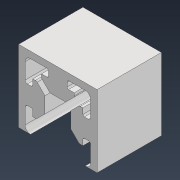
# Autodesk Inventor part: Part6
Saved by Autodesk Inventor 2022 (Build 260153000, 153)
## iProperties
Created: 2022-06-24
Part Number: Part6
Material: Generic
Document SubType Name: Modeling
Designer: tecware
Density: 1 g/cm^3
Appearance: Default
Author: tecware
Autodesk Inventor part; units mm, degrees
ref_plane "YZ Plane" through (0, 0, 0) normal (1, 0, 0) x (0, 1, 0)
ref_plane "XZ Plane" through (0, 0, 0) normal (0, 1, 0) x (-1, 0, 0)
ref_plane "XY Plane" through (0, 0, 0) normal (0, 0, 1) x (1, 0, 0)
sketch "Sketch1" plane through (0, 0, 0) normal (0, 0, 1) x (1, 0, 0)
  arc A0 (-1.0546, 0.6324) -> (-0.3475, 0.9253) centre (-1.0546, 1.6324) ccw projected
  line L0 (-1.0546, 0.6324) -> (-1.8676, 0.6324) projected
  arc A1 (-2.0676, 0.8324) -> (-1.8676, 0.6324) centre (-1.8676, 0.8324) ccw projected
  line L1 (-2.0676, 0.8324) -> (-2.0676, 2.6024) projected
  arc A2 (-2.0676, 2.6024) -> (-2.3176, 2.8524) centre (-2.3176, 2.6024) ccw projected
  line L2 (-2.3176, 2.8524) -> (-3.5676, 2.8524) projected
  arc A3 (-3.5676, 2.8524) -> (-4.0676, 2.3524) centre (-3.5676, 2.3524) ccw projected
  line L3 (-4.0676, 2.3524) -> (-4.0676, -2.5676) projected
  arc A4 (-4.0676, -2.5676) -> (-2.5676, -4.0676) centre (-2.5676, -2.5676) ccw projected
  line L4 (-2.5676, -4.0676) -> (2.3524, -4.0676) projected
  arc A5 (2.3524, -4.0676) -> (2.8524, -3.5676) centre (2.3524, -3.5676) ccw projected
  line L5 (2.8524, -3.5676) -> (2.8524, -2.3176) projected
  arc A6 (2.8524, -2.3176) -> (2.6024, -2.0676) centre (2.6024, -2.3176) ccw projected
  line L6 (2.6024, -2.0676) -> (0.8324, -2.0676) projected
  arc A7 (0.6324, -1.8676) -> (0.8324, -2.0676) centre (0.8324, -1.8676) ccw projected
  line L7 (0.6324, -1.8676) -> (0.6324, -1.0546) projected
  arc A8 (0.9253, -0.3475) -> (0.6324, -1.0546) centre (1.6324, -1.0546) ccw projected
  line L8 (0.9253, -0.3475) -> (4.0676, 2.7948) projected
  arc A9 (4.0676, 2.7948) -> (5.6798, 2.2912) centre (5.9324, 5.9324) ccw projected
  line L9 (5.6798, 2.2912) -> (5.9324, 2.491) projected
  line L10 (5.9324, 2.491) -> (6.1851, 2.2912) projected
  arc A10 (6.1851, 2.2912) -> (7.7973, 2.7948) centre (5.9324, 5.9324) ccw projected
  line L11 (7.7973, 2.7948) -> (10.9395, -0.3475) projected
  arc A11 (11.2324, -1.0546) -> (10.9395, -0.3475) centre (10.2324, -1.0546) ccw projected
  line L12 (11.2324, -1.0546) -> (11.2324, -1.8676) projected
  arc A12 (11.0324, -2.0676) -> (11.2324, -1.8676) centre (11.0324, -1.8676) ccw projected
  line L13 (11.0324, -2.0676) -> (9.2624, -2.0676) projected
  arc A13 (9.2624, -2.0676) -> (9.0124, -2.3176) centre (9.2624, -2.3176) ccw projected
  line L14 (9.0124, -2.3176) -> (9.0124, -3.5676) projected
  arc A14 (9.0124, -3.5676) -> (9.5124, -4.0676) centre (9.5124, -3.5676) ccw projected
  line L15 (9.5124, -4.0676) -> (14.4324, -4.0676) projected
  arc A15 (14.4324, -4.0676) -> (15.9324, -2.5676) centre (14.4324, -2.5676) ccw projected
  line L16 (15.9324, -2.5676) -> (15.9324, 2.3524) projected
  arc A16 (15.9324, 2.3524) -> (15.4324, 2.8524) centre (15.4324, 2.3524) ccw projected
  line L17 (15.4324, 2.8524) -> (14.1824, 2.8524) projected
  arc A17 (14.1824, 2.8524) -> (13.9324, 2.6024) centre (14.1824, 2.6024) ccw projected
  line L18 (13.9324, 2.6024) -> (13.9324, 0.8324) projected
  arc A18 (13.7324, 0.6324) -> (13.9324, 0.8324) centre (13.7324, 0.8324) ccw projected
  line L19 (13.7324, 0.6324) -> (12.9194, 0.6324) projected
  arc A19 (12.2123, 0.9253) -> (12.9194, 0.6324) centre (12.9194, 1.6324) ccw projected
  line L20 (12.2123, 0.9253) -> (9.0701, 4.0676) projected
  arc A20 (9.0701, 4.0676) -> (9.5737, 5.6798) centre (5.9324, 5.9324) ccw projected
  line L21 (9.5737, 5.6798) -> (9.3739, 5.9324) projected
  line L22 (9.3739, 5.9324) -> (9.5739, 6.1824) projected
  arc A21 (9.5739, 6.1824) -> (9.0701, 7.7973) centre (5.9324, 5.9324) ccw projected
  line L23 (9.0701, 7.7973) -> (12.2123, 10.9395) projected
  arc A22 (12.9194, 11.2324) -> (12.2123, 10.9395) centre (12.9194, 10.2324) ccw projected
  line L24 (12.9194, 11.2324) -> (13.7324, 11.2324) projected
  arc A23 (13.9324, 11.0324) -> (13.7324, 11.2324) centre (13.7324, 11.0324) ccw projected
  line L25 (13.9324, 11.0324) -> (13.9324, 9.2624) projected
  arc A24 (13.9324, 9.2624) -> (14.1824, 9.0124) centre (14.1824, 9.2624) ccw projected
  line L26 (14.1824, 9.0124) -> (15.4324, 9.0124) projected
  arc A25 (15.4324, 9.0124) -> (15.9324, 9.5124) centre (15.4324, 9.5124) ccw projected
  line L27 (15.9324, 9.5124) -> (15.9324, 14.4324) projected
  arc A26 (15.9324, 14.4324) -> (14.4324, 15.9324) centre (14.4324, 14.4324) ccw projected
  line L28 (14.4324, 15.9324) -> (9.5124, 15.9324) projected
  arc A27 (9.5124, 15.9324) -> (9.0124, 15.4324) centre (9.5124, 15.4324) ccw projected
  line L29 (9.0124, 15.4324) -> (9.0124, 14.1824) projected
  arc A28 (9.0124, 14.1824) -> (9.2624, 13.9324) centre (9.2624, 14.1824) ccw projected
  line L30 (9.2624, 13.9324) -> (11.0324, 13.9324) projected
  arc A29 (11.2324, 13.7324) -> (11.0324, 13.9324) centre (11.0324, 13.7324) ccw projected
  line L31 (11.2324, 13.7324) -> (11.2324, 12.9194) projected
  arc A30 (10.9395, 12.2123) -> (11.2324, 12.9194) centre (10.2324, 12.9194) ccw projected
  line L32 (10.9395, 12.2123) -> (7.7973, 9.0701) projected
  arc A31 (7.7973, 9.0701) -> (6.1824, 9.5739) centre (5.9324, 5.9324) ccw projected
  line L33 (6.1824, 9.5739) -> (5.9324, 9.3739) projected
  line L34 (5.9324, 9.3739) -> (5.6824, 9.5739) projected
  arc A32 (5.6824, 9.5739) -> (4.0676, 9.0701) centre (5.9324, 5.9324) ccw projected
  line L35 (4.0676, 9.0701) -> (0.9253, 12.2123) projected
  arc A33 (0.6324, 12.9194) -> (0.9253, 12.2123) centre (1.6324, 12.9194) ccw projected
  line L36 (0.6324, 12.9194) -> (0.6324, 13.7324) projected
  arc A34 (0.8324, 13.9324) -> (0.6324, 13.7324) centre (0.8324, 13.7324) ccw projected
  line L37 (0.8324, 13.9324) -> (2.6024, 13.9324) projected
  arc A35 (2.6024, 13.9324) -> (2.8524, 14.1824) centre (2.6024, 14.1824) ccw projected
  line L38 (2.8524, 14.1824) -> (2.8524, 15.4324) projected
  arc A36 (2.8524, 15.4324) -> (2.3524, 15.9324) centre (2.3524, 15.4324) ccw projected
  line L39 (2.3524, 15.9324) -> (-2.5676, 15.9324) projected
  arc A37 (-2.5676, 15.9324) -> (-4.0676, 14.4324) centre (-2.5676, 14.4324) ccw projected
  line L40 (-4.0676, 14.4324) -> (-4.0676, 9.5124) projected
  arc A38 (-4.0676, 9.5124) -> (-3.5676, 9.0124) centre (-3.5676, 9.5124) ccw projected
  line L41 (-3.5676, 9.0124) -> (-2.3176, 9.0124) projected
  arc A39 (-2.3176, 9.0124) -> (-2.0676, 9.2624) centre (-2.3176, 9.2624) ccw projected
  line L42 (-2.0676, 9.2624) -> (-2.0676, 11.0324) projected
  arc A40 (-1.8676, 11.2324) -> (-2.0676, 11.0324) centre (-1.8676, 11.0324) ccw projected
  line L43 (-1.8676, 11.2324) -> (-1.0546, 11.2324) projected
  arc A41 (-0.3475, 10.9395) -> (-1.0546, 11.2324) centre (-1.0546, 10.2324) ccw projected
  line L44 (-0.3475, 10.9395) -> (2.7948, 7.7973) projected
  arc A42 (2.7948, 7.7973) -> (2.291, 6.1824) centre (5.9324, 5.9324) ccw projected
  line L45 (2.291, 6.1824) -> (2.491, 5.9324) projected
  line L46 (2.491, 5.9324) -> (2.2912, 5.6798) projected
  arc A43 (2.2912, 5.6798) -> (2.7948, 4.0676) centre (5.9324, 5.9324) ccw projected
  line L47 (2.7948, 4.0676) -> (-0.3475, 0.9253) projected
  circle A44 centre (5.9324, 5.9324) radius 2.5 projected
  line L48 (-1.0546, 11.0324) -> (-1.8676, 11.0324)
  line L49 (-1.8676, 11.0324) -> (-1.8676, 9.2624)
  arc A45 (-2.3176, 8.8124) -> (-1.8676, 9.2624) centre (-2.3176, 9.2624) ccw
  line L50 (-2.3176, 8.8124) -> (-3.5676, 8.8124)
  arc A46 (-4.2676, 9.5124) -> (-3.5676, 8.8124) centre (-3.5676, 9.5124) ccw
  line L51 (-4.2676, 9.5124) -> (-4.2676, 14.4324)
  arc A47 (-2.5676, 16.1324) -> (-4.2676, 14.4324) centre (-2.5676, 14.4324) ccw
  line L52 (-2.5676, 16.1324) -> (2.3524, 16.1324)
  arc A48 (3.0524, 15.4324) -> (2.3524, 16.1324) centre (2.3524, 15.4324) ccw
  line L53 (3.0524, 15.4324) -> (3.0524, 14.1824)
  arc A49 (2.6024, 13.7324) -> (3.0524, 14.1824) centre (2.6024, 14.1824) ccw
  line L54 (2.6024, 13.7324) -> (0.8324, 13.7324)
  line L55 (0.8324, 13.7324) -> (0.8324, 12.9194)
  arc A50 (0.8324, 12.9194) -> (1.0667, 12.3537) centre (1.6324, 12.9194) ccw
  line L56 (1.0667, 12.3537) -> (4.1014, 9.3191)
  arc A51 (5.7474, 9.778) -> (4.1014, 9.3191) centre (5.9324, 5.9324) ccw
  line L57 (5.7474, 9.778) -> (5.9324, 9.63)
  line L58 (5.9324, 9.63) -> (6.1174, 9.778)
  arc A52 (7.7635, 9.3191) -> (6.1174, 9.778) centre (5.9324, 5.9324) ccw
  line L59 (7.7635, 9.3191) -> (10.7981, 12.3537)
  arc A53 (10.7981, 12.3537) -> (11.0324, 12.9194) centre (10.2324, 12.9194) ccw
  line L60 (11.0324, 12.9194) -> (11.0324, 13.7324)
  line L61 (11.0324, 13.7324) -> (9.2624, 13.7324)
  arc A54 (8.8124, 14.1824) -> (9.2624, 13.7324) centre (9.2624, 14.1824) ccw
  line L62 (8.8124, 14.1824) -> (8.8124, 15.4324)
  arc A55 (9.5124, 16.1324) -> (8.8124, 15.4324) centre (9.5124, 15.4324) ccw
  line L63 (9.5124, 16.1324) -> (14.4324, 16.1324)
  arc A56 (16.1324, 14.4324) -> (14.4324, 16.1324) centre (14.4324, 14.4324) ccw
  line L64 (16.1324, 14.4324) -> (16.1324, 9.5124)
  arc A57 (15.4324, 8.8124) -> (16.1324, 9.5124) centre (15.4324, 9.5124) ccw
  line L65 (15.4324, 8.8124) -> (14.1824, 8.8124)
  arc A58 (13.7324, 9.2624) -> (14.1824, 8.8124) centre (14.1824, 9.2624) ccw
  line L66 (13.7324, 9.2624) -> (13.7324, 11.0324)
  line L67 (13.7324, 11.0324) -> (12.9194, 11.0324)
  arc A59 (12.9194, 11.0324) -> (12.3537, 10.7981) centre (12.9194, 10.2324) ccw
  line L68 (12.3537, 10.7981) -> (9.3191, 7.7635)
  arc A60 (9.778, 6.1174) -> (9.3191, 7.7635) centre (5.9324, 5.9324) ccw
  line L69 (9.778, 6.1174) -> (9.6294, 5.9317)
  line L70 (9.6294, 5.9317) -> (9.7778, 5.7441)
  arc A61 (9.3191, 4.1014) -> (9.7778, 5.7441) centre (5.9324, 5.9324) ccw
  line L71 (9.3191, 4.1014) -> (12.3537, 1.0667)
  arc A62 (12.3537, 1.0667) -> (12.9194, 0.8324) centre (12.9194, 1.6324) ccw
  line L72 (12.9194, 0.8324) -> (13.7324, 0.8324)
  line L73 (13.7324, 0.8324) -> (13.7324, 2.6024)
  arc A63 (14.1824, 3.0524) -> (13.7324, 2.6024) centre (14.1824, 2.6024) ccw
  line L74 (14.1824, 3.0524) -> (15.4324, 3.0524)
  arc A64 (16.1324, 2.3524) -> (15.4324, 3.0524) centre (15.4324, 2.3524) ccw
  line L75 (16.1324, 2.3524) -> (16.1324, -2.5676)
  arc A65 (14.4324, -4.2676) -> (16.1324, -2.5676) centre (14.4324, -2.5676) ccw
  line L76 (14.4324, -4.2676) -> (9.5124, -4.2676)
  arc A66 (8.8124, -3.5676) -> (9.5124, -4.2676) centre (9.5124, -3.5676) ccw
  line L77 (8.8124, -3.5676) -> (8.8124, -2.3176)
  arc A67 (9.2624, -1.8676) -> (8.8124, -2.3176) centre (9.2624, -2.3176) ccw
  line L78 (9.2624, -1.8676) -> (11.0324, -1.8676)
  line L79 (11.0324, -1.8676) -> (11.0324, -1.0546)
  arc A68 (11.0324, -1.0546) -> (10.7981, -0.4889) centre (10.2324, -1.0546) ccw
  line L80 (10.7981, -0.4889) -> (7.7635, 2.5457)
  arc A69 (6.1208, 2.087) -> (7.7635, 2.5457) centre (5.9324, 5.9324) ccw
  line L81 (6.1208, 2.087) -> (5.9324, 2.236)
  line L82 (5.9324, 2.236) -> (5.7441, 2.087)
  arc A70 (4.1014, 2.5457) -> (5.7441, 2.087) centre (5.9324, 5.9324) ccw
  line L83 (4.1014, 2.5457) -> (1.0667, -0.4889)
  arc A71 (1.0667, -0.4889) -> (0.8324, -1.0546) centre (1.6324, -1.0546) ccw
  line L84 (0.8324, -1.0546) -> (0.8324, -1.8676)
  line L85 (0.8324, -1.8676) -> (2.6024, -1.8676)
  arc A72 (3.0524, -2.3176) -> (2.6024, -1.8676) centre (2.6024, -2.3176) ccw
  line L86 (3.0524, -2.3176) -> (3.0524, -3.5676)
  arc A73 (2.3524, -4.2676) -> (3.0524, -3.5676) centre (2.3524, -3.5676) ccw
  line L87 (2.3524, -4.2676) -> (-2.5676, -4.2676)
  arc A74 (-4.2676, -2.5676) -> (-2.5676, -4.2676) centre (-2.5676, -2.5676) ccw
  line L88 (-4.2676, -2.5676) -> (-4.2676, 2.3524)
  arc A75 (-3.5676, 3.0524) -> (-4.2676, 2.3524) centre (-3.5676, 2.3524) ccw
  line L89 (-3.5676, 3.0524) -> (-2.3176, 3.0524)
  arc A76 (-1.8676, 2.6024) -> (-2.3176, 3.0524) centre (-2.3176, 2.6024) ccw
  line L90 (-1.8676, 2.6024) -> (-1.8676, 0.8324)
  line L91 (-1.8676, 0.8324) -> (-1.0546, 0.8324)
  arc A77 (-1.0546, 0.8324) -> (-0.4889, 1.0667) centre (-1.0546, 1.6324) ccw
  line L92 (-0.4889, 1.0667) -> (2.5457, 4.1014)
  arc A78 (2.087, 5.7441) -> (2.5457, 4.1014) centre (5.9324, 5.9324) ccw
  line L93 (2.087, 5.7441) -> (2.2354, 5.9317)
  line L94 (2.2354, 5.9317) -> (2.0869, 6.1174)
  arc A79 (2.5457, 7.7635) -> (2.0869, 6.1174) centre (5.9324, 5.9324) ccw
  line L95 (2.5457, 7.7635) -> (-0.4889, 10.7981)
  arc A80 (-0.4889, 10.7981) -> (-1.0546, 11.0324) centre (-1.0546, 10.2324) ccw
  line L96 (-4.2676, -4.2676) -> (-6.2676, -4.2676)
  line L97 (-6.2676, -4.2676) -> (-6.2676, 18.1324)
  line L98 (-6.2676, 18.1324) -> (18.1324, 18.1324)
  line L99 (18.1324, 18.1324) -> (18.1324, -4.2676)
  line L100 (18.1324, -4.2676) -> (14.4324, -4.2676)
  line L101 (-4.2676, -4.2676) -> (-2.5676, -4.2676)
  line L102 (5.9324, 5.9324) -> (1.9324, 5.9324) construction
  line L103 (1.9324, 8.3768) -> (1.9324, 3.4881)
  line L104 (9.9324, 8.3768) -> (9.9324, 3.4881)
  line L105 (8.3768, 9.9324) -> (3.4881, 9.9324)
  line L106 (5.9324, 5.9324) -> (5.9324, 9.9324) construction
  point P0 (0, 0)
  dimension "d0" = 0.2
  dimension "d1" = 2
  dimension "d2" = 22.4
  dimension "d3" = 24.4
  dimension "d4" = 4
  dimension "d5" = 4
  constraints: 118 end point, 72 point on circle, 36 centre point, 3 point on line, 1 midpoint, 83 other
  measures "d0" radial gap between concentric circles of A41 A80
  measures "d1" distance of L96.start L96.end
  measures "d2" distance of L96.end L97.end
  measures "d3" distance of L97.end L98.end
  measures "d4" distance of L102.start L102.end
  measures "d5" distance of L102.start L106.end
extrude "Extrusion1" add sketch "Sketch1" along normal blind 20 contours A80 L95 L103 L92 A77 L91 L90 A76 L89 A75 L88 A74 L101 L96 L97 L98 L99 L100 A65 L75 A64 L74 A63 L73 L72 A62 L71 L104 L68 A59 L67 L66 A58 L65 A57 L64 A56 L63 A55 L62 A54 L61 L60 A53 L59 L105 L56 A50 L55 L54 A49 L53 A48 L52 A47 L51 A46 L50 A45 L49 L48
body "Solid1"
